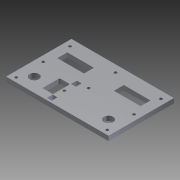
# Autodesk Inventor part: carro x lado motor pieza 4
Saved by Autodesk Inventor 2012 (Build 160160000, 160)
## iProperties
Created: 2014-12-17
Part Number: carro x lado motor pieza 4
Material: Default
Document SubType Name: Modeling
Designer: PRINCIPAL
Density: 1 g/cm^3
Author: PRINCIPAL
Autodesk Inventor part; units mm, degrees
ref_plane "YZ Plane" through (0, 0, 0) normal (1, 0, 0) x (0, 1, 0)
ref_plane "XZ Plane" through (0, 0, 0) normal (0, 1, 0) x (-1, 0, 0)
ref_plane "XY Plane" through (0, 0, 0) normal (0, 0, 1) x (1, 0, 0)
sketch "Boceto1" plane through (0, 0, 0) normal (0, 0, 1) x (1, 0, 0)
  arc A0 (-116.1173, 21.3488) -> (-117.6673, 19.7988) centre (-116.1173, 19.7988) ccw
  arc A1 (-117.6673, 19.7988) -> (-116.1173, 18.2488) centre (-116.1173, 19.7988) ccw
  arc A2 (-116.1173, 18.2488) -> (-114.5673, 19.7988) centre (-116.1173, 19.7988) ccw
  arc A3 (-114.5673, 19.7988) -> (-116.1173, 21.3488) centre (-116.1173, 19.7988) ccw
  arc A4 (-67.1173, 21.3488) -> (-68.6673, 19.7988) centre (-67.1173, 19.7988) ccw
  arc A5 (-68.6673, 19.7988) -> (-67.1173, 18.2488) centre (-67.1173, 19.7988) ccw
  arc A6 (-67.1173, 18.2488) -> (-65.5673, 19.7988) centre (-67.1173, 19.7988) ccw
  arc A7 (-65.5673, 19.7988) -> (-67.1173, 21.3488) centre (-67.1173, 19.7988) ccw
  arc A8 (-18.1173, 21.3488) -> (-19.6673, 19.7988) centre (-18.1173, 19.7988) ccw
  arc A9 (-19.6673, 19.7988) -> (-18.1173, 18.2488) centre (-18.1173, 19.7988) ccw
  arc A10 (-18.1173, 18.2488) -> (-16.5673, 19.7988) centre (-18.1173, 19.7988) ccw
  arc A11 (-16.5673, 19.7988) -> (-18.1173, 21.3488) centre (-18.1173, 19.7988) ccw
  arc A12 (-18.1173, -7.6512) -> (-19.6673, -9.2012) centre (-18.1173, -9.2012) ccw
  arc A13 (-19.6673, -9.2012) -> (-18.1173, -10.7512) centre (-18.1173, -9.2012) ccw
  arc A14 (-18.1173, -10.7512) -> (-16.5673, -9.2012) centre (-18.1173, -9.2012) ccw
  arc A15 (-16.5673, -9.2012) -> (-18.1173, -7.6512) centre (-18.1173, -9.2012) ccw
  arc A16 (-67.1173, -7.6512) -> (-68.6673, -9.2012) centre (-67.1173, -9.2012) ccw
  arc A17 (-68.6673, -9.2012) -> (-67.1173, -10.7512) centre (-67.1173, -9.2012) ccw
  arc A18 (-67.1173, -10.7512) -> (-65.5673, -9.2012) centre (-67.1173, -9.2012) ccw
  arc A19 (-65.5673, -9.2012) -> (-67.1173, -7.6512) centre (-67.1173, -9.2012) ccw
  arc A20 (-116.1173, -7.6512) -> (-117.6673, -9.2012) centre (-116.1173, -9.2012) ccw
  arc A21 (-117.6673, -9.2012) -> (-116.1173, -10.7512) centre (-116.1173, -9.2012) ccw
  arc A22 (-116.1173, -10.7512) -> (-114.5673, -9.2012) centre (-116.1173, -9.2012) ccw
  arc A23 (-114.5673, -9.2012) -> (-116.1173, -7.6512) centre (-116.1173, -9.2012) ccw
  arc A24 (-116.1173, -36.6512) -> (-117.6673, -38.2012) centre (-116.1173, -38.2012) ccw
  arc A25 (-117.6673, -38.2012) -> (-116.1173, -39.7512) centre (-116.1173, -38.2012) ccw
  arc A26 (-116.1173, -39.7512) -> (-114.5673, -38.2012) centre (-116.1173, -38.2012) ccw
  arc A27 (-114.5673, -38.2012) -> (-116.1173, -36.6512) centre (-116.1173, -38.2012) ccw
  arc A28 (-18.1173, -36.6512) -> (-19.6673, -38.2012) centre (-18.1173, -38.2012) ccw
  arc A29 (-19.6673, -38.2012) -> (-18.1173, -39.7512) centre (-18.1173, -38.2012) ccw
  arc A30 (-18.1173, -39.7512) -> (-16.5673, -38.2012) centre (-18.1173, -38.2012) ccw
  arc A31 (-16.5673, -38.2012) -> (-18.1173, -36.6512) centre (-18.1173, -38.2012) ccw
  arc A32 (-107.1173, -22.7762) -> (-112.0423, -27.7012) centre (-107.1173, -27.7012) ccw
  arc A33 (-112.0423, -27.7012) -> (-107.1173, -32.6262) centre (-107.1173, -27.7012) ccw
  arc A34 (-107.1173, -32.6262) -> (-102.1923, -27.7012) centre (-107.1173, -27.7012) ccw
  arc A35 (-102.1923, -27.7012) -> (-107.1173, -22.7762) centre (-107.1173, -27.7012) ccw
  arc A36 (-27.1173, -22.7762) -> (-32.0423, -27.7012) centre (-27.1173, -27.7012) ccw
  arc A37 (-32.0423, -27.7012) -> (-27.1173, -32.6262) centre (-27.1173, -27.7012) ccw
  arc A38 (-27.1173, -32.6262) -> (-22.1923, -27.7012) centre (-27.1173, -27.7012) ccw
  arc A39 (-22.1923, -27.7012) -> (-27.1173, -22.7762) centre (-27.1173, -27.7012) ccw
  arc A40 (-77.8673, -23.1512) -> (-79.4173, -24.7012) centre (-77.8673, -24.7012) ccw
  arc A41 (-79.4173, -24.7012) -> (-77.8673, -26.2512) centre (-77.8673, -24.7012) ccw
  arc A42 (-77.8673, -26.2512) -> (-76.3173, -24.7012) centre (-77.8673, -24.7012) ccw
  arc A43 (-76.3173, -24.7012) -> (-77.8673, -23.1512) centre (-77.8673, -24.7012) ccw
  line L0 (-111.9673, 1.9488) -> (-83.2673, 1.9488)
  line L1 (-83.2673, 1.9488) -> (-83.2673, 12.6488)
  line L2 (-83.2673, 12.6488) -> (-111.9673, 12.6488)
  line L3 (-111.9673, 12.6488) -> (-111.9673, 1.9488)
  line L4 (-50.9673, 12.6488) -> (-50.9673, 1.9488)
  line L5 (-50.9673, 1.9488) -> (-22.2673, 1.9488)
  line L6 (-22.2673, 1.9488) -> (-22.2673, 12.6488)
  line L7 (-22.2673, 12.6488) -> (-50.9673, 12.6488)
  line L8 (-80.7673, -16.563) -> (-81.6794, -15.5552)
  line L9 (-81.6794, -15.5552) -> (-91.0552, -15.5552)
  line L10 (-91.0552, -15.5552) -> (-91.9673, -16.563)
  line L11 (-91.9673, -16.563) -> (-91.9673, -34.0068)
  line L12 (-91.9673, -34.0068) -> (-80.7673, -34.0068)
  line L13 (-80.7673, -34.0068) -> (-80.7673, -16.563)
  line L14 (-11.9023, 27.5138) -> (-122.3323, 27.5138)
  line L15 (-122.3323, 27.5138) -> (-122.3323, -42.9162)
  line L16 (-122.3323, -42.9162) -> (-11.9023, -42.9162)
  line L17 (-11.9023, -42.9162) -> (-11.9023, 27.5138)
  line L18 (-75.3023, -14.7662) -> (-75.3023, -8.6362)
  line L19 (-75.3023, -8.6362) -> (-80.4323, -8.6362)
  line L20 (-80.4323, -8.6362) -> (-80.4323, -14.7662)
  line L21 (-80.4323, -14.7662) -> (-75.3023, -14.7662)
  line L22 (-80.4323, -34.6362) -> (-80.4323, -40.7662)
  line L23 (-80.4323, -40.7662) -> (-75.3023, -40.7662)
  line L24 (-75.3023, -40.7662) -> (-75.3023, -34.6362)
  line L25 (-75.3023, -34.6362) -> (-80.4323, -34.6362)
  point P0 (0, 0)
  constraints: 88 point on circle, 52 end point, 44 centre point
extrude "Extrusión1" add sketch "Boceto1" along normal blind 5
